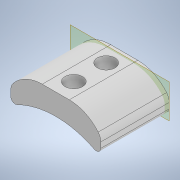
# Autodesk Inventor part: PipeHolder
Saved by Autodesk Inventor 2020.2 (Build 242310000, 310)
## iProperties
Created: 2019-12-08
Part Number: PipeHolder
Material: Generic
Document SubType Name: Modeling
Designer: Paul Lefeuvre
Density: 1 g/cm^3
Appearance: Default
Author: Paul Lefeuvre
Autodesk Inventor part; units mm, degrees
ref_plane "YZ Plane" through (0, 0, 0) normal (1, 0, 0) x (0, 1, 0)
ref_plane "XZ Plane" through (0, 0, 0) normal (0, 1, 0) x (-1, 0, 0)
ref_plane "XY Plane" through (0, 0, 0) normal (0, 0, 1) x (1, 0, 0)
sketch "Sketch1" plane through (0, 0, 0) normal (0, 0, 1) x (1, 0, 0)
  circle A0 centre (0, 0) radius 37.5 construction
  circle A1 centre (0, 0) radius 38.1
  line L0 (0, 0) -> (0, 82.8508) construction
  line L1 (-6, 47.5) -> (6, 47.5)
  line L2 (20, 35.8331) -> (20, 38.2923)
  line L3 (-20, 35.8331) -> (-20, 38.2923)
  arc A2 (-6, 47.5) -> (-18.8366, 41.4986) centre (-6, 30.7709) ccw
  arc A3 (18.8366, 41.4986) -> (6, 47.5) centre (6, 30.7709) ccw
  arc A4 (-18.8366, 41.4986) -> (-20, 38.2923) centre (-15, 38.2923) ccw
  arc A5 (20, 38.2923) -> (18.8366, 41.4986) centre (15, 38.2923) ccw
  arc A6 (17.1022, 34.0459) -> (-17.1022, 34.0459) centre (0, 0) ccw
  arc A7 (-20, 35.8331) -> (-17.1022, 34.0459) centre (-18, 35.8331) ccw
  arc A8 (17.1022, 34.0459) -> (20, 35.8331) centre (18, 35.8331) ccw
  point P0 (20, 32.4285)
  point P1 (20, 39.9285)
  point P2 (-20, 32.4285)
  point P3 (-20, 39.9285)
  point P4 (-17.1022, 34.0459)
  dimension "d0" = 75
  dimension "d1" = 0.6
  dimension "d22" = 12
  dimension "d23" = 6
  dimension "d24" = 47.5
  dimension "d25" = 7.5
  dimension "d26" = 7.5
  dimension "d27" = 40
  dimension "d28" = 20
  dimension "d29" = 5
  dimension "d30" = 2
  constraints: 20 point on circle, 10 tangent, 9 centre point, 8 end point, 4 point on line, 3 vertical, 2 equal radius, 1 coincident, 1 horizontal
  measures "d0" diameter of A0
  measures "d1" radial gap between concentric circles of A0 A1
  measures "d22" distance of L1.start L1.end
  measures "d23" distance from line of L0 L1.start
  measures "d24" distance from line of L0.start L1
  measures "d25" distance of A1.start point (20, 39.929)
  measures "d26" distance of A1.end point (-20, 39.929)
  measures "d27" distance of point (-20, 39.929) point (20, 39.929)
  measures "d28" distance from line of L0 point (-20, 39.929)
  measures "d29" radius of A4
  measures "d30" radius of A7
extrude "Extrusion1" add sketch "Sketch1" along normal blind 30.4 contours A1 A7 L3 A4 A2 L1 A3 A5 L2 A8
sketch "Sketch2" plane through (-6, 47.5, 0) normal (0, 1, 0) x (1, 0, 0)
  line L0 (12, -30.4) -> (0, -30.4) projected
  line L1 (12, 0) -> (12, -30.4) projected
  line L2 (0, -30.4) -> (16.9706, -30.4) construction
  line L3 (12, -30.4) -> (24.8366, -30.4) projected
  line L4 (0, 0) -> (0, -30.4) projected
  line L5 (23.1022, 0) -> (-11.1022, 0) projected
  circle A0 centre (6, -22.4) radius 3.9
  circle A1 centre (6, -8) radius 3.9
  point P0 (6, 0)
  dimension "d34" = 7.8
  dimension "d35" = 7.8
  dimension "d38" = 12
  dimension "d39" = 6
  dimension "d40" = 6
  dimension "d41" = 8
  dimension "d42" = 8
  constraints: 2 centre point, 2 end point, 1 horizontal
  measures "d34" diameter of A0
  measures "d35" diameter of A1
  measures "d38" distance of L1.start L4.start
  measures "d39" distance from line of L4 A1.centre
  measures "d40" distance from line of L4 A0.centre
  measures "d41" distance from line of L0 A0.centre
  measures "d42" distance from line of L5 A1.centre
extrude "Extrusion2" cut sketch "Sketch2" against normal blind 15 contours A0 | A1
ref_plane "Work Plane1" through (0, 0, 2) normal (0, 0, -1) x (-1, 0, 0)
sketch "Sketch3" plane through (0, 0, 2) normal (0, 0, -1) x (-1, 0, 0)
  arc A0 (17.1022, 34.0459) -> (-17.1022, 34.0459) centre (0, 0) ccw projected
  line L0 (-15, 35.023) -> (-15, 36.023)
  line L1 (15, 35.023) -> (15, 36.023)
  line L2 (0, 0) -> (0, 39.8883) construction
  arc A1 (15, 36.023) -> (-15, 36.023) centre (0, 0) ccw
  dimension "d44" = 1
  dimension "d45" = 30
  dimension "d46" = 15
  constraints: 6 end point, 4 point on circle, 3 vertical, 1 centre point, 1 coincident
  measures "d44" distance of L0.end L0.start
  measures "d45" distance of L1.start L0.start
  measures "d46" distance from line of L2 L0.start
extrude "Extrusion3" cut sketch "Sketch3" against normal blind 26.4
equation "\"d23\" = 0.5 * d22"
equation "\"d28\" = 0.5 * d27"
equation "\"d35\" = d34"
equation "\"d39\" = 0.5 * d38"
equation "\"d40\" = 0.5 * d38"
equation "\"d42\" = d41"
equation "\"d46\" = 0.5 * d45"
body "Solid1"
